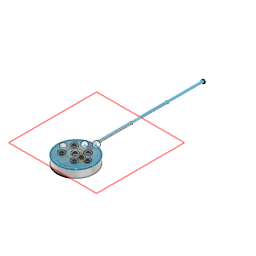
2024_10_14_BlueSubmarineRC v1 (Autodesk Fusion 360 design; units mm, degrees)
Autodesk Fusion 360 part; units mm, degrees
note: some values were not read from the file. Chosen so that the rebuilt part matches the saved one: which bodies a step acts on.
sketch "Sketch1" plane through (0, 0, 0) normal (0, 0, 1) x (1, 0, 0)
sketch "Sketch2" plane through (0, 0, 0) normal (0, 0, 1) x (1, 0, 0)
  circle A0 centre (0.1525, -28.081) radius 24.5522
  line L0 (-11.054, -19.2977) -> (-11.054, -35.9964) construction
  line L1 (-11.054, -35.9964) -> (7.025, -35.9964) construction
  line L2 (7.025, -35.9964) -> (7.025, -19.2977) construction
  line L3 (7.025, -19.2977) -> (-11.054, -19.2977) construction
  circle A1 centre (7.025, -27.6471) radius 8.3493 construction
  line L4 (7.025, -27.6471) -> (-1.3243, -27.6471) construction
  line L5 (7.025, -27.6471) -> (15.3744, -27.6471) construction
  circle A2 centre (15.3744, -27.6471) radius 3.984
  circle A3 centre (-1.3243, -27.6471) radius 3.984
  circle A4 centre (-11.054, -35.9964) radius 3.984
  line L6 (7.025, -19.2977) -> (7.025, -18.2977)
  line L7 (7.025, -35.9964) -> (7.025, -36.9964)
  circle A5 centre (7.025, -36.9964) radius 3.984
  circle A6 centre (7.025, -18.2977) radius 3.984
  circle A7 centre (-11.054, -19.2977) radius 3.984
  circle A8 centre (-6.0235, -10.0208) radius 0.99
  circle A9 centre (-18.4122, -26.606) radius 2.6415
  dimension "d5" = 1
  dimension "d6" = 1
  constraint vertical L0
  constraint perpendicular L0 L1
  constraint perpendicular L1 L2
  constraint perpendicular L0 L3
  constraint midpoint L2 A1.centre
  constraint coincident L2.end A1
  constraint coincident A1.centre L4.start
  constraint coincident A1 L4.end
  constraint perpendicular L2 L4
  constraint coincident A1 L5.end
  constraint perpendicular L2 L5
  constraint coincident L5.end A2.centre
  constraint coincident L4.end A3.centre
  constraint coincident L0.end L1.start
  constraint perpendicular L3 L6
  constraint perpendicular L1 L7
  constraint coincident L7.end A5.centre
  constraint coincident L6.end A6.centre
  constraint coincident L0.start L3.end
  constraint equal A4 A7
  constraint equal A4 A6
  constraint equal A3 A4
  constraint equal A4 A5
  constraint equal A2 A4
  measures "d5" distance of L2.end L6.end
  measures "d6" distance of L1.end L7.end
extrude "Extrude1" add sketch "Sketch2" against normal blind 10 contours A0 | A2 | A3 | A4 | A5 | A6 | A7 | A8 | A9 makes body 1
extrude "Extrude2" cut sketch "Sketch2" against normal blind 2 contours A2 | A3 | A4 | A5 | A6 | A7 bodies 1
extrude "Extrude3" add sketch "Sketch2" along normal blind -2 and the other way blind -1 separate body contours A2 | A3 | A4 | A5 | A6 | A7 makes body 2 at (-7.0898, -19.6944, 0) makes body 3 at (-7.0898, -36.3931, 0) makes body 4 at (10.9892, -37.3931, 0) makes body 5 at (2.6399, -28.0438, 0) makes body 6 at (10.9892, -18.6944, 0) makes body 7 at (19.3386, -28.0438, 0)
sketch "Sketch3" plane through (0, 0, 0) normal (0, 0, 1) x (1, 0, 0)
  line L0 (2.0379, -2.2178) -> (-1.385, -2.2178)
  line L1 (-1.385, -2.2178) -> (-1.385, 46.1297)
  line L2 (-1.385, 46.1297) -> (0.3265, 46.1297)
  line L3 (0.3265, 46.1297) -> (0.3265, -2.2178)
  line L4 (0.3265, 46.1297) -> (0.3265, 94.4772)
  line L5 (0.3265, 94.4772) -> (0.3265, 142.8247)
  line L6 (0.3265, 46.1297) -> (-0.9735, 46.1297)
  line L7 (-0.9735, 46.1297) -> (-0.9735, 94.4772)
  line L8 (-0.9735, 94.4772) -> (0.3265, 94.4772)
  line L9 (0.3265, 94.4772) -> (0.3265, 46.1297)
  line L10 (0.3265, 94.4772) -> (-0.6735, 94.4772)
  line L11 (-0.6735, 94.4772) -> (-0.6735, 142.8247)
  line L12 (-0.6735, 142.8247) -> (0.3265, 142.8247)
  line L13 (0.3265, 142.8247) -> (0.3265, 94.4772)
  line L14 (0.3265, 142.8247) -> (-1.6735, 142.8247)
  line L15 (-1.6735, 142.8247) -> (-1.6735, 143.8247)
  line L16 (-1.6735, 143.8247) -> (0.3265, 143.8247)
  line L17 (0.3265, 143.8247) -> (0.3265, 142.8247)
  dimension "d13" = 1.3
  dimension "d14" = 1
  dimension "d15" = 2
  dimension "d16" = 1
  constraint horizontal L0
  constraint perpendicular L0 L1
  constraint perpendicular L1 L2
  constraint midpoint L0 L3.end
  constraint perpendicular L0 L3
  constraint perpendicular L0 L4
  constraint perpendicular L0 L5
  constraint equal L3 L4
  constraint equal L3 L5
  constraint horizontal L6
  constraint vertical L7
  constraint horizontal L8
  constraint vertical L9
  constraint horizontal L10
  constraint vertical L11
  constraint horizontal L12
  constraint vertical L13
  constraint horizontal L14
  constraint vertical L15
  constraint horizontal L16
  constraint vertical L17
  measures "d13" distance of L2.end L6.end
  measures "d14" distance of L4.end L10.end
  measures "d15" distance of L5.end L14.end
  measures "d16" distance of L5.end L16.end
revolve "Revolve2" add sketch "Sketch3" angle 360 about axis through (0.3265, 46.1297, 0) along (0, 1, 0) separate body contours L0 L1 L2 L3 L6 | L5 L8 L10 L11 L12 L13 L14 makes body 8 at (-1.3828, 13.8981, -0.0853) makes body 9 at (-0.6723, 110.5931, -0.0498)
revolve "Revolve3" add sketch "Sketch3" angle 360 about axis through (0.3265, 46.1297, 0) along (0, 1, 0) separate body contours L2 L4 L6 L7 L8 L9 L10 makes body 10
revolve "Revolve4" add sketch "Sketch3" angle 360 about axis through (0.3265, 142.8247, 0) along (0, -1, 0) contours L12 L14 L15 L16 L17 bodies 9
extrude "Extrude4" cut sketch "Sketch2" against normal blind 1 contours A8 | A9 bodies 1
